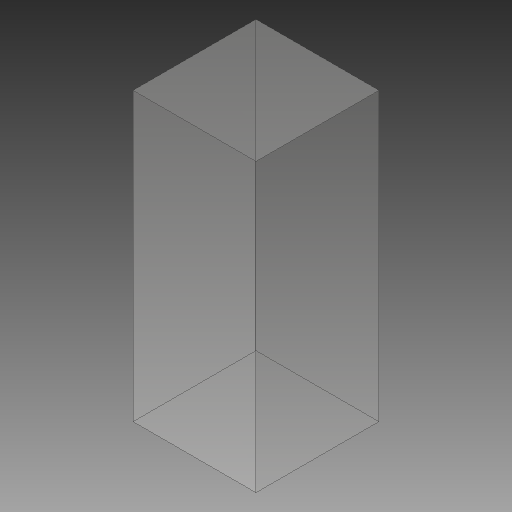
# Autodesk Inventor part: Mold Design1_Part1_WP
Saved by Autodesk Inventor 2018 (Build 220112000, 112)
## iProperties
Created: 2017-12-19
Part Number: Mold Design1_Part1_WP
Material: Generic
Document SubType Name: Modeling
Designer: 238438
Density: 1 g/cm^3
Appearance: Default
Author: 238438
d0: -0.750 in
d1: 0.750 in
d2: 0.750 in
d3: 1.750 in
d4: 1.750 in
d5: 1.500 in
d6: 0.00 deg
Xmin: -0.750 in
Ymin: -1.750 in
Zmin: -0.750 in
Xmax: 0.750 in
Ymax: 1.750 in
Zmax: 0.750 in
Autodesk Inventor part; units mm, degrees
ref_plane "YZ Plane" through (0, 0, 0) normal (1, 0, 0) x (0, 1, 0)
ref_plane "XZ Plane" through (0, 0, 0) normal (0, 1, 0) x (-1, 0, 0)
ref_plane "XY Plane" through (0, 0, 0) normal (0, 0, 1) x (1, 0, 0)
sketch "Sketch1" plane through (0, 0, -19.05) normal (0, 0, 1) x (1, 0, 0)
  line L0 (-19.05, 44.45) -> (19.05, 44.45)
  line L1 (19.05, 44.45) -> (19.05, -44.45)
  line L2 (19.05, -44.45) -> (-19.05, -44.45)
  line L3 (-19.05, -44.45) -> (-19.05, 44.45)
  point P0 (0, 0)
  dimension "d1" = 19.05
  dimension "d2" = 19.05
  dimension "d3" = 44.45
  dimension "d4" = 44.45
  constraints: 8 end point, 2 parallel, 1 horizontal, 1 perpendicular, 1 other
  measures "d1" distance from line of L3 point (0, 0)
  measures "d2" distance from line of L1 point (0, 0)
  measures "d3" distance from line of L2 point (0, 0)
  measures "d4" distance from line of L0 point (0, 0)
extrude "Extrusion1" add sketch "Sketch1" along normal blind 38.1
equation "\"d1\" = -Xmin"
equation "\"d2\" = Xmax"
equation "\"d3\" = -Ymin"
equation "\"d4\" = Ymax"
equation "\"d5\" = Zmax - Zmin"
equation "\"Xmin\" = -19.05"
equation "\"Ymin\" = -44.45"
equation "\"Zmin\" = -19.05"
equation "\"Xmax\" = 19.05"
equation "\"Ymax\" = 44.45"
equation "\"Zmax\" = 19.05"
body "Solid1"
